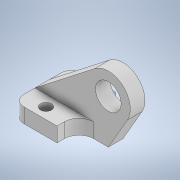
# Autodesk Inventor part: AnchorBase
Saved by Autodesk Inventor 2022.2 (Build 262287030, 287C)
## iProperties
Created: 2023-04-24
Part Number: AnchorBase
Material: Generic
Document SubType Name: Modeling
Designer: jak27277
Density: 1 g/cm^3
Appearance: Default
Author: jak27277
Autodesk Inventor part; units mm, degrees
ref_plane "YZ Plane" through (0, 0, 0) normal (1, 0, 0) x (0, 1, 0)
ref_plane "XZ Plane" through (0, 0, 0) normal (0, 1, 0) x (-1, 0, 0)
ref_plane "XY Plane" through (0, 0, 0) normal (0, 0, 1) x (1, 0, 0)
sketch "Sketch1" plane through (0, 0, 0) normal (0, 0, 1) x (1, 0, 0)
  circle A0 centre (0, 0) radius 22.225
  arc A1 (32.9956, -19.05) -> (-23.4434, 30.0336) centre (0, 0) ccw
  line L0 (32.9956, -19.05) -> (0, -76.2)
  line L1 (0, -76.2) -> (-127, -76.2)
  line L2 (-127, -76.2) -> (-127, -50.8)
  line L3 (-127, -50.8) -> (-23.4434, 30.0336)
  dimension "d0" = 44.45
  dimension "d1" = 38.1
  dimension "d2" = 76.2
  dimension "d3" = 127
  dimension "d4" = 25.4
  constraints: 8 end point, 2 centre point, 2 coincident, 2 point on circle, 2 tangent, 1 horizontal, 1 perpendicular, 1 vertical alignment
  measures "d0" diameter of A0
  measures "d1" radius of A1
  measures "d2" distance from line of L1 point (0, 0)
  measures "d3" distance of L0.end L1.end
  measures "d4" distance of L1.end L2.end
extrude "Extrusion1" add sketch "Sketch1" along normal mid plane 25.4
sketch "Sketch2" plane through (-127, -76.2, 12.7) normal (0, -1, 0) x (1, 0, 0)
  line L0 (0, -25.4) -> (0, 0) construction
  line L1 (0, -12.7) -> (165.1, -12.7) construction
  line L2 (165.1, -25.4) -> (165.1, 0) construction
  line L3 (0, -12.7) -> (0, 19.05)
  line L4 (19.05, 38.1) -> (76.2, 38.1)
  line L5 (76.2, 38.1) -> (76.2, 25.4)
  line L6 (76.2, 25.4) -> (76.2, 0.0039) construction
  arc A0 (76.2, 25.4) -> (101.6, 0) centre (101.6, 25.4) ccw
  line L7 (101.6, 0) -> (0, 0)
  circle A1 centre (38.1, 19.05) radius 9.525
  arc A2 (19.05, 38.1) -> (0, 19.05) centre (19.05, 19.05) ccw
  line L8 (0, 0) -> (0, -25.4) construction
  line L9 (0, -12.7) -> (0, -44.45)
  line L10 (19.05, -63.5) -> (76.2, -63.5)
  line L11 (76.2, -63.5) -> (76.2, -50.8)
  line L12 (76.2, -50.8) -> (76.2, -25.4039) construction
  arc A3 (101.6, -25.4) -> (76.2, -50.8) centre (101.6, -50.8) ccw
  line L13 (101.6, -25.4) -> (0, -25.4)
  circle A4 centre (38.1, -44.45) radius 9.525
  arc A5 (0, -44.45) -> (19.05, -63.5) centre (19.05, -44.45) ccw
  point P0 (127, -12.7)
  point P1 (0, 38.1)
  point P2 (0, -63.5)
  dimension "d7" = 19.05
  dimension "d8" = 101.6
  dimension "d9" = 19.05
  dimension "d10" = 76.2
  dimension "d11" = 25.4
  dimension "d12" = 19.05
  dimension "d13" = 38.1
  constraints: 24 end point, 12 symmetric about line, 8 point on circle, 8 point on line, 6 centre point, 4 tangent, 2 midpoint, 2 perpendicular, 1 horizontal, 3 other
  measures "d7" radius of A2
  measures "d8" distance between parallel lines of L10 L4
  measures "d9" distance from line of A1.centre L4
  measures "d10" distance between parallel lines of L3 L6
  measures "d11" radius of A0
  measures "d12" diameter of A1
  measures "d13" distance from line of A1.centre L3
extrude "Extrusion2" add sketch "Sketch2" against normal blind 25.4
body "Solid1"
